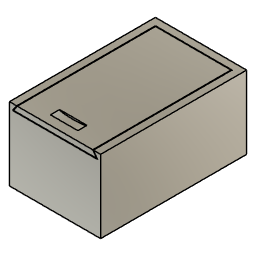
slide_Lid_WithBox v1 (Autodesk Fusion 360 design; units mm, degrees)
Autodesk Fusion 360 part; units mm, degrees
sketch "Sketch1" plane through (0, 0, 0) normal (0, 0, 1) x (1, 0, 0) in component "Box"
box "BoxPrimitive1" add length 80 width 50 height 40 placed x (0, 1, 0) y (-1, 0, 0) z (0, 0, 1) at (50, 0, 0) makes body 1 in component "Box"
shell "Shell1" thickness 4 removed faces 1 at (16.6667, 26.6667, 40) on bodies 1 in component "Box"
sketch "Sketch2" plane through (0, 0, 0) normal (0, -1, 0) x (1, 0, 0) in component "Box"
  line L0 (0, 40) -> (0, 0)
  line L1 (0, 0) -> (50, 0)
  line L2 (50, 0) -> (50, 40)
  line L3 (50, 40) -> (0, 40)
  line L4 (46, 40) -> (48.2943, 36.7234)
  line L5 (46, 40) -> (50, 40) construction
  line L6 (25, 40) -> (25, 36.7234) construction
  line L7 (25, 36.7234) -> (48.2943, 36.7234)
  line L8 (25, 36.7234) -> (1.7057, 36.7234)
  line L9 (4, 40) -> (1.7057, 36.7234)
  point P0 (4, 40)
  point P1 (46, 40)
  dimension "d7" = 55
  dimension "d8" = 4
  constraint horizontal L5
  constraint coincident P1 L4.start
  constraint coincident L2.end L3.start
  constraint midpoint L3 L6.start
  constraint perpendicular L3 L6
  constraint horizontal L4.end L6.end
  constraint symmetric P1 L6 P0
  constraint symmetric L4.end L6 L8.end
  constraint symmetric L7.start L6 L8.start
  measures "d7" angle of L4 L5
  measures "d8" distance of P1 L4.end
extrude "Extrude1" cut sketch "Sketch2" against normal up to surface (76 mm away) contours L3 L4 L7 L8 L9 bodies 1 in component "Box"
sketch "Lid" plane through (0, 0, 0) normal (0, -1, 0) x (1, 0, 0) in component "Lid"
  line L0 (1.7057, 36.7234) -> (4, 40)
  line L1 (4, 40) -> (0, 40)
  line L2 (0, 40) -> (0, 0)
  line L3 (0, 0) -> (50, 0)
  line L4 (50, 0) -> (50, 40)
  line L5 (50, 40) -> (46, 40)
  line L6 (46, 40) -> (48.2943, 36.7234)
  line L7 (48.2943, 36.7234) -> (1.7057, 36.7234)
  line L8 (1.7057, 36.7234) -> (4, 40)
  line L9 (48.2943, 36.7234) -> (1.7057, 36.7234)
  line L10 (46, 40) -> (48.2943, 36.7234)
  line L11 (4, 40) -> (46, 40)
  line L12 (50, 40.25) -> (45.5198, 40.25)
  line L13 (45.5198, 40.25) -> (47.8141, 36.9734)
  line L14 (47.8141, 36.9734) -> (2.1859, 36.9734)
  line L15 (2.1859, 36.9734) -> (4.4802, 40.25)
  line L16 (4.4802, 40.25) -> (0, 40.25)
  line L17 (45.6948, 40) -> (4.3052, 40)
  dimension "d11" = 0.25
  constraint coincident L13 L17.start
  constraint coincident L11 L17.start
  constraint coincident L11 L17.end
  constraint coincident L15 L17.end
extrude "Extrude1'" add sketch "Lid" against normal up to surface (75.75 mm away) separate body contours L11 L13 L14 L15 L17 makes body 2 in component "Lid"
sketch "Sketch1 (2)" plane through (0, 0, 0) normal (0, -1, 0) x (1, 0, 0)
  line L0 (47.8141, 36.9734) -> (45.6948, 40)
  line L1 (45.6948, 40) -> (4.3052, 40)
  line L2 (4.3052, 40) -> (2.1859, 36.9734)
  line L3 (2.1859, 36.9734) -> (47.8141, 36.9734)
  ellipse E0 centre (25, 40) end of major axis (32.5, 40) minor radius 1
  line L4 (17.5, 40) -> (32.5, 40) construction
  line L5 (25, 39) -> (25, 41) construction
  dimension "d19" = 15
  dimension "d20" = 2
  constraint coincident E0 L4.start
  constraint coincident E0 L4.end
  constraint coincident E0 L5.start
  constraint coincident E0 L5.end
  constraint midpoint L1 E0.centre
  constraint parallel L1 L4
  measures "d19" distance of E0
extrude "Extrude2" cut sketch "Sketch1 (2)" along normal blind 5 from surface at -10 contours L1 E0 picked at (23.0364, 39.7937) bodies 2 in component "Lid"
component "Box" placed x (1, 0, 0) y (0, 1, 0) z (0, 0, 1) at (0, 0, 0)
component "Lid" placed x (1, 0, 0) y (0, 1, 0) z (0, 0, 1) at (0, 0, 0)
equation "d1 = length"
equation "d2 = width"
equation "d3 = height"
equation "d6 = thickness"
equation "d8 = thickness"
equation "d11 = clearence"
equation "d12 = clearence"
equation "length = 80 mm"
equation "width = 50 mm"
equation "height = 40 mm"
equation "thickness = 4 mm"
equation "clearence = 0.25 mm"
